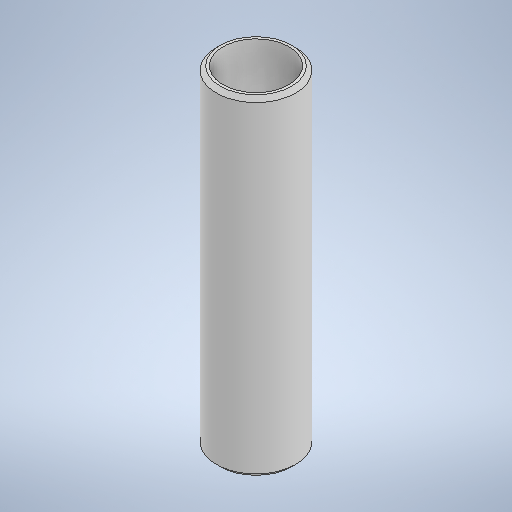
# Autodesk Inventor part: 26-10-211
Saved by Autodesk Inventor 2025.2 (Build 292293000, 293)
## iProperties
Category: 5
Manager: 3
Company: 4
Created: 2024-11-14
Part Number: 26-10-211
Material: Generic
Document SubType Name: Modeling
Designer: Zvonko.Gabric
Density: 1 g/cm^3
Appearance: Default
Project: 10
Cost Center: 13
Catalog Web Link: 15
Description: Guide sleeve,
Vendor: 14
Engineer: 11
Authority: 12
Stock Number: 8
Author: Zvonko.Gabric
Title: Compression spring
Subject: 2
Keywords: 6
Comments: 7
Revision Number: 9
Autodesk Inventor part; units mm, degrees
ref_plane "YZ Plane" through (0, 0, 0) normal (1, 0, 0) x (0, 1, 0)
ref_plane "XZ Plane" through (0, 0, 0) normal (0, 1, 0) x (-1, 0, 0)
ref_plane "XY Plane" through (0, 0, 0) normal (0, 0, 1) x (1, 0, 0)
sketch "Sketch1" plane through (0, 0, 0) normal (0, 1, 0) x (-1, 0, 0)
  circle A0 centre (0, 0) radius 3
  circle A1 centre (0, 0) radius 2.75
  dimension "d0" = 6
  dimension "d1" = 5.5
  constraints: 2 centre point, 1 coincident
  measures "d0" diameter of A0
  measures "d1" diameter of A1
extrude "Extrusion1" add sketch "Sketch1" along normal blind 25 contours A0 | A1
chamfer "Chamfer1" distance 0.3 angle 45 2 edges at (3, 25, 0) (3, 0, 0) measured on face at (-2.9612, 8.3333, -0.4812)
sketch "Sketch2" plane through (0, 25, 0) normal (0, 1, 0) x (1, 0, 0)
  circle A0 centre (0, 0) radius 2.5
  dimension "d7" = 5
  constraints: 1 centre point, 1 coincident
  measures "d7" diameter of A0
extrude "Extrusion2" cut sketch "Sketch2" against normal blind 50
body "Solid1"
